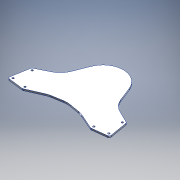
# Autodesk Inventor part: Ball Stop
Saved by Autodesk Inventor 2019.4 (Build 234330000, 330)
## iProperties
Created: 2020-01-06
Part Number: Ball Stop
Material: Aluminum 6061
Document SubType Name: Modeling
Designer: admin
Density: 2.7 g/cm^3
Appearance: Aluminum - Flat
Author: admin
Autodesk Inventor part; units mm, degrees
ref_plane "YZ Plane" through (0, 0, 0) normal (1, 0, 0) x (0, 1, 0)
ref_plane "XZ Plane" through (0, 0, 0) normal (0, 1, 0) x (-1, 0, 0)
ref_plane "XY Plane" through (0, 0, 0) normal (0, 0, 1) x (1, 0, 0)
sketch "Sketch1" plane through (0, 0, 0) normal (0, 1, 0) x (-1, 0, 0)
  line L0 (0, 64.6605) -> (51.1872, 78.4039)
  line L1 (51.1872, 78.4039) -> (80.8718, 117.2674)
  line L2 (80.8718, 117.2674) -> (139.8816, 146.2193)
  line L3 (139.8816, 146.2193) -> (150, 206.2555)
  line L4 (150, 206.2555) -> (100.2877, 211.9786)
  line L5 (100.2877, 211.9786) -> (47.3509, 188.9648)
  line L6 (47.3509, 188.9648) -> (0, 181.018)
  line L7 (0, 181.018) -> (0, 64.6605) construction
  line L8 (0, 64.6605) -> (-51.1872, 78.4039)
  line L9 (-51.1872, 78.4039) -> (-80.8718, 117.2674)
  line L10 (-80.8718, 117.2674) -> (-139.8816, 146.2193)
  line L11 (-139.8816, 146.2193) -> (-150, 206.2555)
  line L12 (-150, 206.2555) -> (-100.2877, 211.9786)
  line L13 (-100.2877, 211.9786) -> (-47.3509, 188.9648)
  line L14 (-47.3509, 188.9648) -> (0, 181.018)
  line L15 (0, 313.5337) -> (0, 181.018)
  dimension "d0" = 150
  constraints: 32 end point, 6 symmetric about line, 2 vertical, 1 other
  measures "d0" distance from line of L7 L3.end
extrude "Extrusion1" add sketch "Sketch1" along normal blind 5
sketch "Sketch2" plane through (0, 5, 0) normal (0, 1, 0) x (1, 0, 0)
  line L0 (0, -64.6605) -> (-51.1872, -78.4039) projected
  line L1 (-51.1872, -78.4039) -> (-80.8718, -117.2674) projected
  line L2 (-80.8718, -117.2674) -> (-139.8816, -146.2193) projected
  line L3 (-139.8816, -146.2193) -> (-150, -206.2555) projected
  line L4 (-150, -206.2555) -> (-100.2877, -211.9786) projected
  line L5 (-100.2877, -211.9786) -> (-47.3509, -188.9648) projected
  line L6 (-47.3509, -188.9648) -> (0, -181.018) projected
  line L7 (0, -181.018) -> (47.3509, -188.9648) projected
  line L8 (47.3509, -188.9648) -> (100.2877, -211.9786) projected
  line L9 (100.2877, -211.9786) -> (150, -206.2555) projected
  line L10 (150, -206.2555) -> (139.8816, -146.2193) projected
  line L11 (139.8816, -146.2193) -> (80.8718, -117.2674) projected
  line L12 (80.8718, -117.2674) -> (51.1872, -78.4039) projected
  line L13 (51.1872, -78.4039) -> (0, -64.6605) projected
  line L14 (-143.7123, -199.0333) -> (-135.6116, -150.9694) construction
  line L15 (-134.1112, -148.9576) -> (-77.6128, -121.2378)
  line L16 (-77.6128, -121.2378) -> (-48.2469, -82.7915)
  line L17 (-48.2469, -82.7915) -> (0, -69.8375)
  line L18 (0, -69.8375) -> (48.2469, -82.7915)
  line L19 (48.2469, -82.7915) -> (77.6128, -121.2378)
  line L20 (77.6128, -121.2378) -> (135.3772, -149.5788)
  line L21 (135.3772, -149.5788) -> (144.1939, -201.8909)
  line L22 (144.1939, -201.8909) -> (101.0497, -206.8578)
  line L23 (101.0497, -206.8578) -> (48.7826, -184.1352)
  line L24 (48.7826, -184.1352) -> (0, -175.9481)
  line L25 (0, -175.9481) -> (-48.7826, -184.1352)
  line L26 (-48.7826, -184.1352) -> (-100.3725, -206.5634)
  line L27 (-101.7834, -206.7733) -> (-141.315, -202.2223) construction
  arc A0 (-143.7123, -199.0333) -> (-141.315, -202.2223) centre (-141.0005, -199.4904) ccw
  arc A1 (-101.7834, -206.7733) -> (-100.3725, -206.5634) centre (-101.4689, -204.0414) ccw
  arc A2 (-134.1112, -148.9576) -> (-135.6116, -150.9694) centre (-132.8999, -151.4264) ccw
  circle A3 centre (-101.4689, -204.0414) radius 2.75
  circle A4 centre (-141.0005, -199.4904) radius 2.75
  circle A5 centre (-132.8999, -151.4264) radius 2.75
  point P0 (0, 0)
  dimension "d3" = 5
  dimension "d4" = 2.75
  dimension "d5" = 2.75
  dimension "d6" = 5.5
  dimension "d7" = 5.5
  dimension "d8" = 5.5
  constraints: 28 end point, 6 centre point, 6 point on circle, 6 tangent, 3 coincident, 1 equal radius, 13 other
  measures "d3" distance between parallel lines of L3 L14
  measures "d4" radius of A0
  measures "d5" radius of A2
  measures "d6" diameter of A3
  measures "d7" diameter of A4
  measures "d8" diameter of A5
extrude "Extrusion2" cut sketch "Sketch2" against normal through all contours A4 A0 | A3 A1 | A5 A2
mirror "Mirror1" about plane through (0, 0, 0) normal (1, 0, 0) of "Extrusion2"
fillet "Fillet1" radius 5 6 edges at (100.2877, 2.5, 211.9786) (150, 2.5, 206.2555) (139.8816, 2.5, 146.2193) (-100.2877, 2.5, 211.9786) (-150, 2.5, 206.2555) (-139.8816, 2.5, 146.2193)
fillet "Fillet2" radius 60 3 edges at (-47.3509, 2.5, 188.9648) (0, 2.5, 181.018) (47.3509, 2.5, 188.9648)
fillet "Fillet3" radius 60 3 edges at (51.1872, 2.5, 78.4039) (0, 2.5, 64.6605) (-51.1872, 2.5, 78.4039)
fillet "Fillet4" radius 60 2 edges at (80.8718, 2.5, 117.2674) (-80.8718, 2.5, 117.2674)
body "Solid1"
